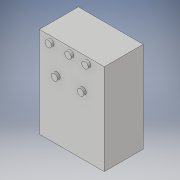
# Autodesk Inventor part: subsystem1
Saved by Autodesk Inventor 2019 (Build 230136000, 136)
## iProperties
Created: 2020-02-19
Part Number: subsystem1
Material: Generic
Document SubType Name: Modeling
Designer: Ridham Sawhney
Density: 1 g/cm^3
Appearance: Default
Author: Ridham Sawhney
Autodesk Inventor part; units mm, degrees
ref_plane "YZ Plane" through (0, 0, 0) normal (1, 0, 0) x (0, 1, 0)
ref_plane "XZ Plane" through (0, 0, 0) normal (0, 1, 0) x (-1, 0, 0)
ref_plane "XY Plane" through (0, 0, 0) normal (0, 0, 1) x (1, 0, 0)
sketch "Sketch1" plane through (0, 0, 0) normal (0, 0, 1) x (1, 0, 0)
  line L0 (0, 0) -> (-50, 0)
  line L1 (-50, 0) -> (-50, 70)
  line L2 (-50, 70) -> (0, 70)
  line L3 (0, 70) -> (0, 0)
  dimension "d0" = 50
  dimension "d1" = 70
  constraints: 8 end point, 2 parallel, 1 horizontal, 1 perpendicular
  measures "d0" distance of L1.end L2.end
  measures "d1" distance of L0.end L1.end
extrude "Extrusion1" add sketch "Sketch1" against normal blind 30
sketch "Sketch2" plane through (0, 0, 0) normal (0, 0, 1) x (1, 0, 0)
  circle A0 centre (-41.2091, 65.6547) radius 2.5
  line L0 (-41.2091, 65.6547) -> (-12.3103, 65.6547)
  circle A1 centre (-25.9431, 65.6547) radius 2.5
  circle A2 centre (-12.8739, 65.6547) radius 2.5
  circle A3 centre (-36.4759, 45.7872) radius 2.5
  line L1 (-36.4759, 45.7872) -> (-11.1478, 45.7872)
  circle A4 centre (-16.3262, 45.7872) radius 2.5
  point P0 (0, 0)
  dimension "d4" = 5
  dimension "d5" = 5
  dimension "d6" = 5
  dimension "d7" = 5
  dimension "d8" = 5
  constraints: 5 centre point, 4 end point, 3 point on line, 2 horizontal
  measures "d4" diameter of A0
  measures "d5" diameter of A1
  measures "d6" diameter of A2
  measures "d7" diameter of A3
  measures "d8" diameter of A4
extrude "Extrusion2" add sketch "Sketch2" along normal blind 2
body "Solid1"
